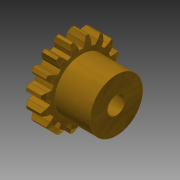
# Autodesk Inventor part: Zahnrad Messing z16
Saved by Autodesk Inventor 2017.3 (Build 213256000, 256)
## iProperties
Category: PARTsolutions
Company: MAEDLER
Created: 2018-08-20
Part Number: Zahnrad Messing z16
Material: Messing, weicher Gelbton, geschweißt
Catalog Web Link: www.cadenas.de
Description: Stzr Messing Ms58-Spur Gears, Brass, Helical Tooth Right Hand, with one-sided hub
Vendor: MAEDLER
Document SubType Name: Modeling
Designer: psadmin
Manufacturer: MAEDLER
Mass: 1.5 g
Surface Area: 2.95369 cm^2
Volume: 0.192618 cm^3
Density: 7.78743 g/cm^3
Appearance: Schweißnaht - Messing
PSOL_IDENT_0: {$CADENAS_DATA\23d-libs\maedler\antriebselemente\stirnzahnraeder\stirnzahnraeder_messing\stzr_messin
PSOL_IDENT_1: g_ms58.prj},204 {VTYP=3D},{NB=Stzr Messing Ms58 26101600},{LINA=Stzr Messing Ms58 26101600},{NN=Stzr
PSOL_IDENT_2: Messing Ms58},{DATE=03.08.2018 09:08:56},{GEOMDATE=26.07.2018 09:15:44},{VERSION=},{LINEID=230},{WB
PSOL_IDENT_3: VAR=},{WBNUMERIC=}  {NB=Stzr Messing Ms58 26101600},{LINA=Stzr Messing Ms58 26101600},{KT=DUMMY},{AR
PSOL_IDENT_4: TNR=26101600},{WST=Messing (Ms58)},{M=0.5},{Z=16},{PDF=PDF Katalogseite},{B1=2.0},{DA=9.00},{D=8.00}
PSOL_IDENT_5: ,{NL=4},{ND=6},{B=2.00},{MD=0.8},{GEW=1.500}
NN: Stzr Messing Ms58
NT: Spur Gears, Brass, Helical Tooth Right Hand, with one-sided hub
NB: Stzr Messing Ms58 26101600
NBSYN: Stzr Messing Ms58 $ARTNR.
LINA: Stzr Messing Ms58 26101600
ARTNR: 26101600
WST: Messing (Ms58)
M: 0.5
Z: 16
PDF: PDF Katalogseite
B1: 2
DA: 9
D: 8
NL: 4
ND: 6
B: 2
MD: 0.8
GEW: 1.5
SUPPLIER: MAEDLER
ARTICLENO: Stzr Messing Ms58 26101600
BOMINFO: Stzr Messing Ms58 26101600
CREATOR: CADENAS GmbH
Title: Stzr Messing Ms58 26101600
Author: Cadenas PARTsolutions
Comments: Spur Gears, Brass, Helical Tooth Right Hand, with one-sided hub
Autodesk Inventor part; units mm, degrees
ref_plane "YZ Plane" through (0, 0, 0) normal (1, 0, 0) x (0, 1, 0)
ref_plane "XZ Plane" through (0, 0, 0) normal (0, 1, 0) x (-1, 0, 0)
ref_plane "XY Plane" through (0, 0, 0) normal (0, 0, 1) x (1, 0, 0)
sketch "Skizze_1" plane through (0, 0, 0) normal (0, 0, 1) x (1, 0, 0)
  line L0 (6, 0) -> (0, 0)
  line L1 (0, 1) -> (6, 1)
  line L2 (6, 1) -> (6, 3)
  line L3 (6, 3) -> (2, 3)
  line L4 (2, 3) -> (2, 4)
  line L5 (2, 4) -> (1, 6.7475)
  line L6 (1, 6.7475) -> (0, 4)
  line L7 (0, 4) -> (0, 1)
  constraints: 16 end point
revolve "Revolution1" add sketch "Skizze_1" angle 360 about axis through (6, 0, 0) along (1, 0, 0)
sketch "Skizze_2" plane through (2, 0, 0) normal (1, 0, 0) x (0, 0, -1)
  circle A0 centre (0, 0) radius 13.5
  arc A1 (-4.443, -0.7138) -> (-4.378, -1.0408) centre (0, 0) ccw
  line L0 (-4.378, -1.0408) -> (-3.8318, -1.1476)
  line L1 (-3.8318, -1.1476) -> (-3.3143, -1.125)
  arc A2 (-3.3143, -1.125) -> (-3.1391, -1.548) centre (0, 0) ccw
  line L2 (-3.1391, -1.548) -> (-3.521, -1.898)
  line L3 (-3.521, -1.898) -> (-3.8316, -2.3598)
  arc A3 (-3.8316, -2.3598) -> (-3.6465, -2.6369) centre (0, 0) ccw
  line L4 (-3.6465, -2.6369) -> (-3.101, -2.5267)
  line L5 (-3.101, -2.5267) -> (-2.6314, -2.3077)
  arc A4 (-2.6314, -2.3077) -> (-2.3077, -2.6314) centre (0, 0) ccw
  line L6 (-2.3077, -2.6314) -> (-2.5267, -3.101)
  line L7 (-2.5267, -3.101) -> (-2.6369, -3.6465)
  arc A5 (-2.6369, -3.6465) -> (-2.3598, -3.8316) centre (0, 0) ccw
  line L8 (-2.3598, -3.8316) -> (-1.898, -3.521)
  line L9 (-1.898, -3.521) -> (-1.548, -3.1391)
  arc A6 (-1.548, -3.1391) -> (-1.125, -3.3143) centre (0, 0) ccw
  line L10 (-1.125, -3.3143) -> (-1.1476, -3.8318)
  line L11 (-1.1476, -3.8318) -> (-1.0408, -4.378)
  arc A7 (-1.0408, -4.378) -> (-0.7138, -4.443) centre (0, 0) ccw
  line L12 (-0.7138, -4.443) -> (-0.4061, -3.9793)
  line L13 (-0.4061, -3.9793) -> (-0.2289, -3.4925)
  arc A8 (-0.2289, -3.4925) -> (0.2289, -3.4925) centre (0, 0) ccw
  line L14 (0.2289, -3.4925) -> (0.4061, -3.9793)
  line L15 (0.4061, -3.9793) -> (0.7138, -4.443)
  arc A9 (0.7138, -4.443) -> (1.0408, -4.378) centre (0, 0) ccw
  line L16 (1.0408, -4.378) -> (1.1476, -3.8318)
  line L17 (1.1476, -3.8318) -> (1.125, -3.3143)
  arc A10 (1.125, -3.3143) -> (1.548, -3.1391) centre (0, 0) ccw
  line L18 (1.548, -3.1391) -> (1.898, -3.521)
  line L19 (1.898, -3.521) -> (2.3598, -3.8316)
  arc A11 (2.3598, -3.8316) -> (2.6369, -3.6465) centre (0, 0) ccw
  line L20 (2.6369, -3.6465) -> (2.5267, -3.101)
  line L21 (2.5267, -3.101) -> (2.3077, -2.6314)
  arc A12 (2.3077, -2.6314) -> (2.6314, -2.3077) centre (0, 0) ccw
  line L22 (2.6314, -2.3077) -> (3.101, -2.5267)
  line L23 (3.101, -2.5267) -> (3.6465, -2.6369)
  arc A13 (3.6465, -2.6369) -> (3.8316, -2.3598) centre (0, 0) ccw
  line L24 (3.8316, -2.3598) -> (3.521, -1.898)
  line L25 (3.521, -1.898) -> (3.1391, -1.548)
  arc A14 (3.1391, -1.548) -> (3.3143, -1.125) centre (0, 0) ccw
  line L26 (3.3143, -1.125) -> (3.8318, -1.1476)
  line L27 (3.8318, -1.1476) -> (4.378, -1.0408)
  arc A15 (4.378, -1.0408) -> (4.443, -0.7138) centre (0, 0) ccw
  line L28 (4.443, -0.7138) -> (3.9793, -0.4061)
  line L29 (3.9793, -0.4061) -> (3.4925, -0.2289)
  arc A16 (3.4925, -0.2289) -> (3.4925, 0.2289) centre (0, 0) ccw
  line L30 (3.4925, 0.2289) -> (3.9793, 0.4061)
  line L31 (3.9793, 0.4061) -> (4.443, 0.7138)
  arc A17 (4.443, 0.7138) -> (4.378, 1.0408) centre (0, 0) ccw
  line L32 (4.378, 1.0408) -> (3.8318, 1.1476)
  line L33 (3.8318, 1.1476) -> (3.3143, 1.125)
  arc A18 (3.3143, 1.125) -> (3.1391, 1.548) centre (0, 0) ccw
  line L34 (3.1391, 1.548) -> (3.521, 1.898)
  line L35 (3.521, 1.898) -> (3.8316, 2.3598)
  arc A19 (3.8316, 2.3598) -> (3.6465, 2.6369) centre (0, 0) ccw
  line L36 (3.6465, 2.6369) -> (3.101, 2.5267)
  line L37 (3.101, 2.5267) -> (2.6314, 2.3077)
  arc A20 (2.6314, 2.3077) -> (2.3077, 2.6314) centre (0, 0) ccw
  line L38 (2.3077, 2.6314) -> (2.5267, 3.101)
  line L39 (2.5267, 3.101) -> (2.6369, 3.6465)
  arc A21 (2.6369, 3.6465) -> (2.3598, 3.8316) centre (0, 0) ccw
  line L40 (2.3598, 3.8316) -> (1.898, 3.521)
  line L41 (1.898, 3.521) -> (1.548, 3.1391)
  arc A22 (1.548, 3.1391) -> (1.125, 3.3143) centre (0, 0) ccw
  line L42 (1.125, 3.3143) -> (1.1476, 3.8318)
  line L43 (1.1476, 3.8318) -> (1.0408, 4.378)
  arc A23 (1.0408, 4.378) -> (0.7138, 4.443) centre (0, 0) ccw
  line L44 (0.7138, 4.443) -> (0.4061, 3.9793)
  line L45 (0.4061, 3.9793) -> (0.2289, 3.4925)
  arc A24 (0.2289, 3.4925) -> (-0.2289, 3.4925) centre (0, 0) ccw
  line L46 (-0.2289, 3.4925) -> (-0.4061, 3.9793)
  line L47 (-0.4061, 3.9793) -> (-0.7138, 4.443)
  arc A25 (-0.7138, 4.443) -> (-1.0408, 4.378) centre (0, 0) ccw
  line L48 (-1.0408, 4.378) -> (-1.1476, 3.8318)
  line L49 (-1.1476, 3.8318) -> (-1.125, 3.3143)
  arc A26 (-1.125, 3.3143) -> (-1.548, 3.1391) centre (0, 0) ccw
  line L50 (-1.548, 3.1391) -> (-1.898, 3.521)
  line L51 (-1.898, 3.521) -> (-2.3598, 3.8316)
  arc A27 (-2.3598, 3.8316) -> (-2.6369, 3.6465) centre (0, 0) ccw
  line L52 (-2.6369, 3.6465) -> (-2.5267, 3.101)
  line L53 (-2.5267, 3.101) -> (-2.3077, 2.6314)
  arc A28 (-2.3077, 2.6314) -> (-2.6314, 2.3077) centre (0, 0) ccw
  line L54 (-2.6314, 2.3077) -> (-3.101, 2.5267)
  line L55 (-3.101, 2.5267) -> (-3.6465, 2.6369)
  arc A29 (-3.6465, 2.6369) -> (-3.8316, 2.3598) centre (0, 0) ccw
  line L56 (-3.8316, 2.3598) -> (-3.521, 1.898)
  line L57 (-3.521, 1.898) -> (-3.1391, 1.548)
  arc A30 (-3.1391, 1.548) -> (-3.3143, 1.125) centre (0, 0) ccw
  line L58 (-3.3143, 1.125) -> (-3.8318, 1.1476)
  line L59 (-3.8318, 1.1476) -> (-4.378, 1.0408)
  arc A31 (-4.378, 1.0408) -> (-4.443, 0.7138) centre (0, 0) ccw
  line L60 (-4.443, 0.7138) -> (-3.9793, 0.4061)
  line L61 (-3.9793, 0.4061) -> (-3.4925, 0.2289)
  arc A32 (-3.4925, 0.2289) -> (-3.4925, -0.2289) centre (0, 0) ccw
  line L62 (-3.4925, -0.2289) -> (-3.9793, -0.4061)
  line L63 (-3.9793, -0.4061) -> (-4.443, -0.7138)
  constraints: 128 end point, 64 point on circle, 33 centre point
extrude "Extrusion1" cut sketch "Skizze_2" along normal mid plane 12
body "Solid1"
